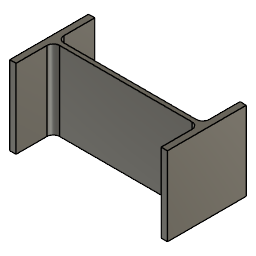
H-200×100×5.5×8 (Autodesk Fusion 360 design; units mm, degrees)
Autodesk Fusion 360 part; units mm, degrees
sketch "スケッチ1" plane through (0, 0, 0) normal (0, 0, 1) x (1, 0, 0)
  line L0 (0, 50) -> (0, -50)
  line L1 (8, -50) -> (8, -10.75)
  line L2 (0, -50) -> (8, -50)
  line L3 (8, 10.75) -> (8, 50)
  line L4 (8, 50) -> (0, 50)
  line L5 (200, -50) -> (200, 50)
  line L6 (192, -10.75) -> (192, -50)
  line L7 (192, -50) -> (200, -50)
  line L8 (184, 2.75) -> (16, 2.75)
  line L9 (16, -2.75) -> (184, -2.75)
  line L10 (192, 50) -> (192, 10.75)
  line L11 (200, 50) -> (192, 50)
  arc A0 (8, 10.75) -> (16, 2.75) centre (16, 10.75) ccw
  arc A1 (16, -2.75) -> (8, -10.75) centre (16, -10.75) ccw
  arc A2 (192, -10.75) -> (184, -2.75) centre (184, -10.75) ccw
  arc A3 (184, 2.75) -> (192, 10.75) centre (184, 10.75) ccw
extrude "押し出し1" add sketch "スケッチ1" along normal blind 100
